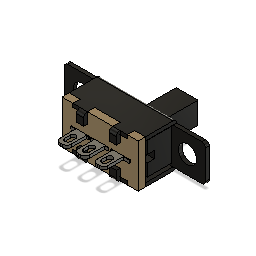
Mini Slide Switch (Autodesk Fusion 360 design; units mm, degrees)
Autodesk Fusion 360 part; units mm, degrees
sketch "Sketch1" plane through (0, 0, 0) normal (0, 1, 0) x (1, 0, 0)
  line L0 (5.25, 2.65) -> (-5.25, 2.65)
  line L1 (-5.25, 2.15) -> (-5.25, -2.65)
  line L2 (-5.25, -2.65) -> (5.25, -2.65)
  line L3 (5.25, -2.65) -> (5.25, 2.15)
  line L4 (5.25, 2.65) -> (-5.25, -2.65) construction
  line L5 (-5.25, 2.65) -> (5.25, -2.65) construction
  line L6 (0, 2.65) -> (9.75, 2.65)
  line L7 (9.75, 2.65) -> (9.75, 2.15)
  line L8 (9.75, 2.15) -> (5.25, 2.15)
  line L9 (0, 2.65) -> (-9.75, 2.65)
  line L10 (-9.75, 2.65) -> (-9.75, 2.15)
  line L11 (-9.75, 2.15) -> (-5.25, 2.15)
  dimension "d1" = 10.5
  dimension "d2" = 5.3
  dimension "d3" = 9.75
  dimension "d4" = 0.5
  dimension "d5" = 9.75
  dimension "d6" = 0.5
  constraint horizontal L0
  constraint perpendicular L0 L1
  constraint parallel L0 L2
  constraint parallel L1 L3
  constraint coincident L4 origin
  constraint coincident L5 origin
  constraint midpoint L0 L6.start
  constraint parallel L0 L6
  constraint perpendicular L6 L7
  constraint perpendicular L3 L8
  constraint parallel L0 L9
  constraint perpendicular L9 L10
  constraint perpendicular L1 L11
  measures "d1" distance of L1.end L2.end
  measures "d2" distance of L0.end L1.end
  measures "d3" distance of L6.start L6.end
  measures "d4" distance of L6.end L7.end
  measures "d5" distance of L6.start L9.end
  measures "d6" distance of L9.end L10.end
extrude "Extrude1" add sketch "Sketch1" along normal blind 6 makes body 1
sketch "Sketch2" plane through (0, 0, -2.65) normal (0, 0, -1) x (-1, 0, 0)
  line L0 (-9.75, 0) -> (9.75, 0)
  line L1 (9.75, 0) -> (9.75, 6)
  line L2 (9.75, 6) -> (-9.75, 6)
  line L3 (-9.75, 6) -> (-9.75, 0)
  line L4 (9.75, 3) -> (7.25, 3)
  line L5 (-9.75, 3) -> (-7.25, 3)
  circle A0 centre (7.25, 3) radius 1.25
  circle A1 centre (-7.25, 3) radius 1.25
  dimension "d9" = 2.5
  dimension "d10" = 2.5
  dimension "d11" = 2.5
  dimension "d12" = 2.5
  constraint midpoint L1 L4.start
  constraint perpendicular L1 L4
  constraint midpoint L3 L5.start
  constraint perpendicular L3 L5
  constraint coincident L4.end A0.centre
  constraint coincident L5.end A1.centre
  measures "d9" distance of L4.start L4.end
  measures "d10" distance of L5.start L5.end
  measures "d11" diameter of A0
  measures "d12" diameter of A1
extrude "Extrude2" cut sketch "Sketch2" against normal blind 5 contours A0 | A1 bodies 1
sketch "Sketch3" plane through (5.25, 0, 0) normal (1, 0, 0) x (0, 0, -1)
  line L0 (-2.65, 0) -> (2.15, 0)
  line L1 (2.15, 0) -> (2.15, 6)
  line L2 (2.15, 6) -> (-2.65, 6)
  line L3 (-2.65, 6) -> (-2.65, 0)
  line L4 (2.15, 5.5) -> (-2.65, 5.5)
  line L5 (-2.65, 0.5) -> (2.15, 0.5)
  constraint coincident L1 L5.end
  constraint coincident L1 L4.start
  constraint coincident L3 L4.end
  constraint coincident L3 L5.start
extrude "Extrude3" cut sketch "Sketch3" against normal blind 16 contours L1 L3 L4 L5 bodies 1
sketch "Sketch4" plane through (0, 0, -2.15) normal (0, 0, 1) x (1, 0, 0)
  circle A0 centre (-7.25, 3) radius 1.25
  circle A1 centre (7.25, 3) radius 1.25
  line L0 (5.25, 0) -> (9.75, 0)
  line L1 (9.75, 0) -> (9.75, 6)
  line L2 (9.75, 6) -> (5.25, 6)
  line L3 (5.25, 6) -> (5.25, 5.5)
  line L4 (5.25, 5.5) -> (-5.25, 5.5)
  line L5 (-5.25, 5.5) -> (-5.25, 6)
  line L6 (-5.25, 6) -> (-9.75, 6)
  line L7 (-9.75, 6) -> (-9.75, 0)
  line L8 (-9.75, 0) -> (-5.25, 0)
  line L9 (-5.25, 0) -> (-5.25, 0.5)
  line L10 (-5.25, 0.5) -> (5.25, 0.5)
  line L11 (5.25, 0.5) -> (5.25, 0)
  line L12 (5.25, 0.5) -> (9.75, 0.5)
  line L13 (5.25, 5.5) -> (9.75, 5.5)
  line L14 (-5.25, 0.5) -> (-9.75, 0.5)
  line L15 (-5.25, 5.5) -> (-9.75, 5.5)
  constraint coincident L10.end L11.start
  constraint coincident L1 L12.end
  constraint perpendicular L1 L12
  constraint coincident L3.end L4.start
  constraint coincident L1 L13.end
  constraint perpendicular L1 L13
  constraint coincident L9.end L10.start
  constraint coincident L7 L14.end
  constraint perpendicular L7 L14
  constraint coincident L4.end L5.start
  constraint coincident L7 L15.end
  constraint perpendicular L7 L15
extrude "Extrude4" cut sketch "Sketch4" against normal blind 15 contours L0 L1 L11 L12 | L7 L8 L9 L14 | L1 L2 L3 L13 | L5 L6 L7 L15 bodies 1
fillet "Fillet2" radius 0.5 4 edges at (-9.75, 0.5, -2.4) (-9.75, 5.5, -2.4) (9.75, 0.5, -2.4) (9.75, 5.5, -2.4) on bodies 1
fillet "Fillet3" radius 0.5 2 edges at (0, 0, -2.65) (0, 6, -2.65) on bodies 1
sketch "Sketch5" plane through (0, 0, -2.65) normal (0, 0, -1) x (-1, 0, 0)
  line L0 (5.25, 5.5) -> (-5.25, 5.5)
  line L1 (-5.25, 5.5) -> (-9.25, 5.5)
  arc A0 (-9.25, 5.5) -> (-9.75, 5) centre (-9.25, 5) ccw
  line L2 (-9.75, 5) -> (-9.75, 1)
  arc A1 (-9.75, 1) -> (-9.25, 0.5) centre (-9.25, 1) ccw
  line L3 (-9.25, 0.5) -> (-5.25, 0.5)
  line L4 (-5.25, 0.5) -> (5.25, 0.5)
  line L5 (5.25, 0.5) -> (9.25, 0.5)
  arc A2 (9.25, 0.5) -> (9.75, 1) centre (9.25, 1) ccw
  line L6 (9.75, 1) -> (9.75, 5)
  arc A3 (9.75, 5) -> (9.25, 5.5) centre (9.25, 5) ccw
  line L7 (9.25, 5.5) -> (5.25, 5.5)
  circle A4 centre (7.25, 3) radius 1.25
  circle A5 centre (-7.25, 3) radius 1.25
  line L8 (-3, 1.5) -> (3, 1.5)
  line L9 (3, 1.5) -> (3, 4.5)
  line L10 (3, 4.5) -> (-3, 4.5)
  line L11 (-3, 4.5) -> (-3, 1.5)
  line L12 (-3, 1.5) -> (3, 4.5) construction
  line L13 (3, 1.5) -> (-3, 4.5) construction
  point P0 (0, 3)
  dimension "d26" = 6
  dimension "d27" = 3
  constraint horizontal L8
  constraint perpendicular L8 L9
  constraint parallel L8 L10
  constraint parallel L9 L11
  constraint coincident L12 P0
  constraint coincident L13 P0
  measures "d26" distance of L9.end L10.end
  measures "d27" distance of L8.end L9.end
extrude "Extrude5" cut sketch "Sketch5" against normal blind 4 contours L8 L9 L10 L11 bodies 1
sketch "Sketch6" plane through (0, 0, 0) normal (0, -1, 0) x (1, 0, 0)
  line L0 (-5.25, -2.15) -> (5.25, -2.15)
  line L1 (5.25, -2.15) -> (5.25, 2.65)
  line L2 (5.25, 2.65) -> (-5.25, 2.65)
  line L3 (-5.25, 2.65) -> (-5.25, -2.15)
  line L4 (5.25, 2.65) -> (3.75, 2.65)
  line L5 (3.75, 2.65) -> (3.75, 1.65)
  line L6 (3.75, 1.65) -> (5.25, 1.65)
  line L7 (-5.25, 2.65) -> (-5.25, 1.65)
  line L8 (-5.25, 1.65) -> (-3.75, 1.65)
  line L9 (3.75, 2.65) -> (1.75, 2.65)
  line L10 (1.75, 2.65) -> (1.75, 1.65)
  line L11 (-3.75, 1.65) -> (-3.75, 2.65)
  line L12 (-3.75, 2.65) -> (-1.75, 2.65)
  line L13 (-1.75, 2.65) -> (-1.75, 1.65)
  line L14 (1.75, 1.65) -> (-1.75, 1.65)
  dimension "d30" = 1.5
  dimension "d31" = 1
  dimension "d32" = 1
  dimension "d33" = 1.5
  dimension "d34" = 2
  dimension "d35" = 1
  dimension "d36" = 2
  dimension "d37" = 1
  constraint coincident L1.end L2.start
  constraint perpendicular L1 L4
  constraint perpendicular L4 L5
  constraint coincident L1 L6.end
  constraint perpendicular L1 L6
  constraint coincident L2.end L3.start
  constraint perpendicular L2 L7
  constraint perpendicular L3 L8
  constraint perpendicular L5 L9
  constraint perpendicular L9 L10
  constraint coincident L2 L11.end
  constraint perpendicular L2 L11
  constraint perpendicular L11 L12
  constraint perpendicular L2 L13
  measures "d30" distance of L1.end L4.end
  measures "d31" distance of L4.end L5.end
  measures "d32" distance of L2.end L7.end
  measures "d33" distance of L7.end L8.end
  measures "d34" distance of L4.end L9.end
  measures "d35" distance of L9.end L10.end
  measures "d36" distance of L11.end L12.end
  measures "d37" distance of L12.end L13.end
extrude "Extrude6" cut sketch "Sketch6" against normal blind 11 contours L2 L3 L7 L8 L11 | L1 L2 L4 L5 L6 | L2 L10 L13 L14 bodies 1
sketch "Sketch7" plane through (0, 0, 1.65) normal (0, 0, 1) x (1, 0, 0)
  line L0 (-3.75, 0.5) -> (-5.25, 0.5)
  line L1 (-5.25, 0.5) -> (-5.25, 0)
  line L2 (-5.25, 0) -> (-3.75, 0)
  line L3 (-3.75, 0) -> (-3.75, 0.5)
  line L4 (-5.25, 0) -> (5.25, 0)
  line L5 (5.25, 0) -> (5.25, 6)
  line L6 (5.25, 6) -> (-5.25, 6)
  line L7 (-5.25, 6) -> (-5.25, 0)
  line L8 (-3.75, 0) -> (-1.75, 0)
  line L9 (-1.75, 0) -> (-1.75, 0.5)
  line L10 (-1.75, 0.5) -> (-3.75, 0.5)
  line L11 (-3.75, 0.5) -> (-3.75, 0)
  line L12 (0, 0) -> (0, 6)
  line L13 (-5.25, 3) -> (5.25, 3)
  line L14 (-1.75, 6) -> (-1.75, 5.5)
  line L15 (-1.75, 5.5) -> (-3.75, 5.5)
  line L16 (-3.75, 5.5) -> (-3.75, 6)
  line L17 (1.75, 0.5) -> (3.75, 0.5)
  line L18 (1.75, 0) -> (1.75, 0.5)
  line L19 (3.75, 0.5) -> (3.75, 0)
  line L20 (1.75, 5.5) -> (3.75, 5.5)
  line L21 (1.75, 6) -> (1.75, 5.5)
  line L22 (3.75, 5.5) -> (3.75, 6)
  dimension "d40" = 10.5
  dimension "d41" = 6
  dimension "d42" = 2
  constraint horizontal L4
  constraint vertical L5
  constraint horizontal L6
  constraint vertical L7
  constraint coincident L1.end L2.start
  constraint horizontal L8
  constraint vertical L9
  constraint horizontal L10
  constraint vertical L11
  constraint coincident L2.end L3.start
  constraint coincident L12.start origin
  constraint midpoint L6 L12.end
  constraint midpoint L7 L13.start
  constraint midpoint L5 L13.end
  constraint symmetric L2.end L13 L16.end
  constraint symmetric L8.end L13 L14.start
  constraint symmetric L9.end L13 L14.end
  constraint symmetric L0.start L13 L15.end
  constraint symmetric L2.end L12 L19.end
  constraint symmetric L8.end L12 L18.start
  constraint symmetric L9.end L12 L17.start
  constraint symmetric L0.start L12 L17.end
  constraint symmetric L12 L14.start L21.start
  constraint symmetric L12 L14.end L20.start
  constraint symmetric L12 L15.end L20.end
  constraint symmetric L12 L16.end L22.end
  measures "d40" distance of L1.end L4.end
  measures "d41" distance of L1.end L6.end
  measures "d42" distance of L2.end L8.end
extrude "Extrude7" add sketch "Sketch7" along normal blind 1 separate body contours L0 L1 L2 L3 L4 L7 L11 | L0 L4 L7 L9 L10 L12 L13 | L6 L7 L12 L13 L14 L15 L16 | L4 L5 L12 L13 L17 L18 L19 | L5 L6 L12 L13 L20 L21 L22 makes body 2
sketch "Sketch8" plane through (0, 0, 2.65) normal (0, 0, 1) x (1, 0, 0)
  line L0 (-1.75, 0) -> (-1.75, 0.5)
  line L1 (-1.75, 0.5) -> (-3.75, 0.5)
  line L2 (-3.75, 0.5) -> (-3.75, 0)
  line L3 (-3.75, 0) -> (-1.75, 0)
  line L4 (-1.75, 0) -> (-2.75, 0)
  line L5 (-2.75, 0) -> (-2.75, 1.5)
  line L6 (-2.75, 1.5) -> (-1.75, 1.5)
  line L7 (-1.75, 1.5) -> (-1.75, 0)
  line L8 (0, 0) -> (0, 6)
  line L9 (0, 3) -> (-5, 3)
  line L10 (-1.75, 4.5) -> (-1.75, 6)
  line L11 (-2.75, 4.5) -> (-1.75, 4.5)
  line L12 (-2.75, 6) -> (-2.75, 4.5)
  line L13 (-1.75, 6) -> (-2.75, 6)
  line L14 (1.75, 1.5) -> (1.75, 0)
  line L15 (2.75, 1.5) -> (1.75, 1.5)
  line L16 (2.75, 0) -> (2.75, 1.5)
  line L17 (1.75, 0) -> (2.75, 0)
  line L18 (2.75, 4.5) -> (1.75, 4.5)
  line L19 (1.75, 4.5) -> (1.75, 6)
  line L20 (2.75, 6) -> (2.75, 4.5)
  line L21 (1.75, 6) -> (2.75, 6)
  dimension "d45" = 1.5
  constraint horizontal L4
  constraint vertical L5
  constraint horizontal L6
  constraint vertical L7
  constraint coincident L0.start L3.end
  constraint coincident L8.start origin
  constraint vertical L8
  constraint midpoint L8 L9.start
  constraint perpendicular L8 L9
  constraint symmetric L0.start L9 L10.end
  constraint symmetric L4.end L9 L12.start
  constraint symmetric L5.end L9 L11.start
  constraint symmetric L6.end L9 L10.start
  constraint symmetric L0.start L8 L14.end
  constraint symmetric L4.end L8 L16.start
  constraint symmetric L5.end L8 L15.start
  constraint symmetric L6.end L8 L14.start
  constraint symmetric L8 L10.start L18.end
  constraint symmetric L8 L10.end L19.end
  constraint symmetric L8 L11.start L18.start
  constraint symmetric L8 L12.start L20.start
  measures "d45" distance of L0.start L6.end
extrude "Extrude8" add sketch "Sketch8" along normal blind 0.5 contours L0 L1 L3 L4 L5 L7 | L1 L5 L6 L7 | L10 L11 L12 L13 | L14 L15 L16 L17 | L18 L19 L20 L21 bodies 1
fillet "Fillet4" radius 0.5 4 edges at (-2.25, 0, 3.15) (2.25, 0, 3.15) (2.25, 6, 3.15) (-2.25, 6, 3.15) on bodies 1
sketch "Sketch9" plane through (0, 0, 1.65) normal (0, 0, -1) x (-1, 0, 0)
  line L0 (1.75, 6) -> (-1.75, 6)
  line L1 (-1.75, 6) -> (-1.75, 5.5)
  line L2 (-1.75, 5.5) -> (-3.75, 5.5)
  line L3 (-3.75, 5.5) -> (-3.75, 6)
  line L4 (-3.75, 6) -> (-5.25, 6)
  line L5 (-5.25, 6) -> (-5.25, 0)
  line L6 (-5.25, 0) -> (-3.75, 0)
  line L7 (-3.75, 0) -> (-3.75, 0.5)
  line L8 (-3.75, 0.5) -> (-1.75, 0.5)
  line L9 (-1.75, 0.5) -> (-1.75, 0)
  line L10 (-1.75, 0) -> (1.75, 0)
  line L11 (1.75, 0) -> (1.75, 0.5)
  line L12 (1.75, 0.5) -> (3.75, 0.5)
  line L13 (3.75, 0.5) -> (3.75, 0)
  line L14 (3.75, 0) -> (5.25, 0)
  line L15 (5.25, 0) -> (5.25, 6)
  line L16 (5.25, 6) -> (3.75, 6)
  line L17 (3.75, 6) -> (3.75, 5.5)
  line L18 (3.75, 5.5) -> (1.75, 5.5)
  line L19 (1.75, 5.5) -> (1.75, 6)
  line L20 (0, 0) -> (0, 6)
  line L21 (5.25, 3) -> (-5.25, 3)
  line L22 (-1.2, 2.8) -> (1.2, 2.8)
  line L23 (1.2, 2.8) -> (1.2, 3.2)
  line L24 (1.2, 3.2) -> (-1.2, 3.2)
  line L25 (-1.2, 3.2) -> (-1.2, 2.8)
  line L26 (-1.2, 2.8) -> (1.2, 3.2) construction
  line L27 (1.2, 2.8) -> (-1.2, 3.2) construction
  line L28 (0, 3) -> (-2.54, 3)
  line L29 (-0.0656, 3) -> (2.4744, 3)
  line L30 (1.4744, 2.8) -> (3.4744, 2.8)
  line L31 (3.4744, 2.8) -> (3.4744, 3.2)
  line L32 (3.4744, 3.2) -> (1.4744, 3.2)
  line L33 (1.4744, 3.2) -> (1.4744, 2.8)
  line L34 (1.4744, 2.8) -> (3.4744, 3.2) construction
  line L35 (3.4744, 2.8) -> (1.4744, 3.2) construction
  line L36 (-3.54, 2.8) -> (-1.54, 2.8)
  line L37 (-1.54, 2.8) -> (-1.54, 3.2)
  line L38 (-1.54, 3.2) -> (-3.54, 3.2)
  line L39 (-3.54, 3.2) -> (-3.54, 2.8)
  line L40 (-3.54, 2.8) -> (-1.54, 3.2) construction
  line L41 (-1.54, 2.8) -> (-3.54, 3.2) construction
  line L42 (0, 3) -> (-4.25, 3)
  line L43 (-1.54, 3.2) -> (-4.14, 3.2)
  line L44 (-1.54, 2.8) -> (-4.14, 2.8)
  line L45 (-4.14, 2.8) -> (-4.14, 3.2)
  line L46 (1.4744, 2.8) -> (3.9744, 2.8)
  line L47 (3.9744, 2.8) -> (3.9744, 3.2)
  line L48 (3.9744, 3.2) -> (3.4744, 3.2)
  point P0 (0, 3)
  point P1 (2.4744, 3)
  point P2 (-2.54, 3)
  dimension "d57" = 2.4
  dimension "d58" = 0.4
  dimension "d59" = 2.54
  dimension "d60" = 2.54
  dimension "d61" = 2
  dimension "d62" = 2
  dimension "d63" = 0.4
  dimension "d64" = 4.25
  dimension "d65" = 2.6
  dimension "d66" = 2.5
  constraint coincident L20.start origin
  constraint midpoint L0 L20.end
  constraint midpoint L15 L21.start
  constraint midpoint L5 L21.end
  constraint horizontal L22
  constraint perpendicular L22 L23
  constraint parallel L22 L24
  constraint parallel L23 L25
  constraint coincident L26 P0
  constraint coincident L27 P0
  constraint midpoint L20 P0
  constraint coincident P0 L28.start
  constraint parallel L21 L28
  constraint coincident L21 L29.start
  constraint perpendicular L23 L29
  constraint horizontal L30
  constraint perpendicular L30 L31
  constraint parallel L30 L32
  constraint parallel L31 L33
  constraint coincident L34 P1
  constraint coincident L35 P1
  constraint coincident P1 L29.end
  constraint horizontal L36
  constraint perpendicular L36 L37
  constraint parallel L36 L38
  constraint parallel L37 L39
  constraint coincident L40 P2
  constraint coincident L41 P2
  constraint coincident P2 L28.end
  constraint perpendicular L39 L42
  constraint perpendicular L39 L43
  constraint perpendicular L37 L44
  constraint perpendicular L43 L45
  constraint perpendicular L31 L46
  constraint perpendicular L21 L47
  constraint perpendicular L31 L48
  measures "d57" distance of L23.end L24.end
  measures "d58" distance of L22.end L23.end
  measures "d59" distance of P0 P2
  measures "d60" distance of L29.start P1
  measures "d61" distance of L31.end L32.end
  measures "d62" distance of L37.end L38.end
  measures "d63" distance of L36.end L37.end
  measures "d64" distance of P0 L42.end
  measures "d65" distance of L37.end L43.end
  measures "d66" distance of L30.start L46.end
extrude "Extrude9" cut sketch "Sketch9" against normal blind 2 contours L20 L21 L23 L24 L29 | L20 L21 L24 L25 L28 L29 L42 | L20 L21 L22 L23 L29 | L20 L21 L22 L25 L28 L29 L42 | L21 L29 L31 L32 L33 | L21 L29 L30 L31 L33 L46 | L21 L28 L36 L37 L39 L42 L44 | L21 L28 L37 L38 L39 L42 L43 | L21 L31 L46 L47 | L21 L31 L47 L48 | L21 L39 L42 L44 L45 | L21 L39 L42 L43 L45 bodies 2
sketch "Sketch10" plane through (0, 0, 1.65) normal (0, 0, -1) x (-1, 0, 0)
  line L0 (1.4744, 2.8) -> (1.4744, 3.2)
  line L1 (1.4744, 3.2) -> (3.9744, 3.2)
  line L2 (3.9744, 3.2) -> (3.9744, 2.8)
  line L3 (3.9744, 2.8) -> (1.4744, 2.8)
  line L4 (1.2, 2.8) -> (-1.2, 2.8)
  line L5 (-1.2, 2.8) -> (-1.2, 3.2)
  line L6 (-1.2, 3.2) -> (1.2, 3.2)
  line L7 (1.2, 3.2) -> (1.2, 2.8)
  line L8 (-4.14, 3.2) -> (-1.54, 3.2)
  line L9 (-1.54, 3.2) -> (-1.54, 2.8)
  line L10 (-1.54, 2.8) -> (-4.14, 2.8)
  line L11 (-4.14, 2.8) -> (-4.14, 3.2)
  line L12 (1.75, 6) -> (-1.75, 6)
  line L13 (-1.75, 6) -> (-1.75, 5.5)
  line L14 (-1.75, 5.5) -> (-3.75, 5.5)
  line L15 (-3.75, 5.5) -> (-3.75, 6)
  line L16 (-3.75, 6) -> (-5.25, 6)
  line L17 (-5.25, 6) -> (-5.25, 0)
  line L18 (-5.25, 0) -> (-3.75, 0)
  line L19 (-3.75, 0) -> (-3.75, 0.5)
  line L20 (-3.75, 0.5) -> (-1.75, 0.5)
  line L21 (-1.75, 0.5) -> (-1.75, 0)
  line L22 (-1.75, 0) -> (1.75, 0)
  line L23 (1.75, 0) -> (1.75, 0.5)
  line L24 (1.75, 0.5) -> (3.75, 0.5)
  line L25 (3.75, 0.5) -> (3.75, 0)
  line L26 (3.75, 0) -> (5.25, 0)
  line L27 (5.25, 0) -> (5.25, 6)
  line L28 (5.25, 6) -> (3.75, 6)
  line L29 (3.75, 6) -> (3.75, 5.5)
  line L30 (3.75, 5.5) -> (1.75, 5.5)
  line L31 (1.75, 5.5) -> (1.75, 6)
extrude "Extrude10" add sketch "Sketch10" along normal blind 1 and the other way blind 1.1 separate body contours L0 L1 L2 L3 | L4 L5 L6 L7 | L8 L9 L10 L11 makes body 3 at (-2.3078, 2.8, 1.35) makes body 4 at (0.4, 2.8, 1.35) makes body 5 at (2.4067, 2.8, 2.05)
extrude "Extrude11" cut 2 faces at (-2.3078, 3.0667, 0.65) (3.2733, 3.0667, 0.65) along direction (0, 0, 1) blind 0.2 on bodies 3 5 bodies 3 5
sketch "Sketch11" plane through (0, 3.2, 0) normal (0, 1, 0) x (-1, 0, 0)
  line L0 (-1.2, 2.75) -> (-1.2, 0.65)
  line L1 (-1.2, 0.65) -> (1.2, 0.65)
  line L2 (1.2, 0.65) -> (1.2, 2.75)
  line L3 (1.2, 2.75) -> (-1.2, 2.75)
  line L4 (1.2, 0.65) -> (1.2, 0.85)
  line L5 (1.2, 0.85) -> (-1.2, 0.85)
  arc A0 (-1.2, 0.85) -> (1.2, 0.85) centre (0, 4.35) ccw
  dimension "d75" = 0.2
  constraint coincident L1.end L2.start
  constraint perpendicular L1 L4
  constraint coincident L0 L5.end
  constraint perpendicular L0 L5
  measures "d75" distance of L1.end L4.end
extrude "Extrude12" cut sketch "Sketch11" against normal blind 1.3 contours L0 L1 A0 | L1 L2 L4 A0 bodies 4
sketch "Sketch12" plane through (0, 0, 2.75) normal (0, 0, 1) x (1, 0, 0)
  line L0 (1.2, 3.2) -> (-1.2, 3.2)
  line L1 (-1.2, 3.2) -> (-1.2, 2.8)
  line L2 (-1.2, 2.8) -> (1.2, 2.8)
  line L3 (1.2, 2.8) -> (1.2, 3.2)
  line L4 (0.75, 3.2) -> (-0.75, 3.2)
  line L5 (-0.75, 3.2) -> (-0.75, 2.8)
  line L6 (-0.75, 2.8) -> (0.75, 2.8)
  line L7 (0.75, 2.8) -> (0.75, 3.2)
  line L8 (0.75, 3.2) -> (-0.75, 2.8) construction
  line L9 (-0.75, 3.2) -> (0.75, 2.8) construction
  line L10 (0, 3) -> (2.54, 3)
  line L11 (0, 3) -> (-2.54, 3)
  line L12 (3.29, 3.2) -> (1.79, 3.2)
  line L13 (1.79, 3.2) -> (1.79, 2.8)
  line L14 (1.79, 2.8) -> (3.29, 2.8)
  line L15 (3.29, 2.8) -> (3.29, 3.2)
  line L16 (3.29, 3.2) -> (1.79, 2.8) construction
  line L17 (1.79, 3.2) -> (3.29, 2.8) construction
  line L18 (-1.79, 3.2) -> (-3.29, 3.2)
  line L19 (-3.29, 3.2) -> (-3.29, 2.8)
  line L20 (-3.29, 2.8) -> (-1.79, 2.8)
  line L21 (-1.79, 2.8) -> (-1.79, 3.2)
  line L22 (-1.79, 3.2) -> (-3.29, 2.8) construction
  line L23 (-3.29, 3.2) -> (-1.79, 2.8) construction
  point P0 (0, 3)
  point P1 (2.54, 3)
  point P2 (-2.54, 3)
  dimension "d78" = 1.5
  dimension "d79" = 2.54
  dimension "d80" = 2.54
  dimension "d81" = 1.5
  dimension "d82" = 1.5
  constraint horizontal L4
  constraint perpendicular L4 L5
  constraint parallel L4 L6
  constraint parallel L5 L7
  constraint coincident L8 P0
  constraint coincident L9 P0
  constraint coincident P0 L10.start
  constraint parallel L0 L10
  constraint parallel L10 L11
  constraint horizontal L12
  constraint perpendicular L12 L13
  constraint parallel L12 L14
  constraint parallel L13 L15
  constraint coincident L16 P1
  constraint coincident L17 P1
  constraint coincident P1 L10.end
  constraint horizontal L18
  constraint perpendicular L18 L19
  constraint parallel L18 L20
  constraint parallel L19 L21
  constraint coincident L22 P2
  constraint coincident L23 P2
  constraint coincident P2 L11.end
  measures "d78" distance of L5.end L6.end
  measures "d79" distance of P0 P1
  measures "d80" distance of P0 P2
  measures "d81" distance of L13.end L14.end
  measures "d82" distance of L19.end L20.end
extrude "Extrude13" add sketch "Sketch12" along normal blind 2.7 contours L0 L4 L5 L7 L10 L11 | L2 L5 L6 L7 L10 L11 | L12 L13 L14 L15 | L18 L19 L20 L21 bodies 3 4 5
fillet "Fillet5" radius 0.6 6 edges at (-1.79, 3, 5.45) (-3.29, 3, 5.45) (-0.75, 3, 5.45) (0.75, 3, 5.45) (1.79, 3, 5.45) (3.29, 3, 5.45) on bodies 3 4 5
sketch "Sketch13" plane through (0, 2.8, 0) normal (0, -1, 0) x (1, 0, 0)
  arc A0 (0.75, 4.85) -> (0.15, 5.45) centre (0.15, 4.85) ccw
  line L0 (0.15, 5.45) -> (-0.15, 5.45)
  arc A1 (-0.15, 5.45) -> (-0.75, 4.85) centre (-0.15, 4.85) ccw
  line L1 (-0.75, 4.85) -> (-0.75, 2.75)
  line L2 (-0.75, 2.75) -> (-1.2, 2.75)
  line L3 (-1.2, 2.75) -> (-1.2, 0.85)
  arc A2 (-1.2, 0.85) -> (1.2, 0.85) centre (0, 4.35) ccw
  line L4 (1.2, 0.85) -> (1.2, 2.75)
  line L5 (1.2, 2.75) -> (0.75, 2.75)
  line L6 (0.75, 2.75) -> (0.75, 4.85)
  line L7 (0, 5.45) -> (0, 4.95)
  line L8 (0, 4.95) -> (0, 3.45)
  line L9 (-0.4, 4.55) -> (-0.4025, 3.8514)
  line L10 (0.4, 4.55) -> (0.3975, 3.8486)
  arc A3 (0.4, 4.5472) -> (-0.4, 4.55) centre (0, 4.55) ccw
  arc A4 (-0.4025, 3.8514) -> (0.3975, 3.8486) centre (-0.0025, 3.85) ccw
  line L11 (0, 4.55) -> (2.54, 4.55)
  line L12 (1.27, 4.55) -> (1.27, 3.7407)
  arc A5 (2.94, 4.55) -> (2.14, 4.5472) centre (2.54, 4.55) ccw
  line L13 (2.94, 4.55) -> (2.9425, 3.8514)
  arc A6 (2.1425, 3.8486) -> (2.9425, 3.8514) centre (2.5425, 3.85) ccw
  line L14 (2.14, 4.55) -> (2.1425, 3.8486)
  line L15 (-2.14, 4.55) -> (-2.1425, 3.8486)
  arc A7 (-2.9425, 3.8514) -> (-2.1425, 3.8486) centre (-2.5425, 3.85) ccw
  line L16 (-2.94, 4.55) -> (-2.9425, 3.8514)
  arc A8 (-2.14, 4.5472) -> (-2.94, 4.55) centre (-2.54, 4.55) ccw
  dimension "d88" = 0.5
  dimension "d89" = 0.8
  dimension "d90" = 1.5
  dimension "d91" = 0.8
  dimension "d92" = 2.54
  constraint midpoint L0 L7.start
  constraint perpendicular L0 L7
  constraint coincident L7.end A3
  constraint parallel L7 L8
  constraint coincident L8.end A4
  constraint tangent L9 A4
  constraint coincident L10.start A3
  constraint tangent L10 A4
  constraint coincident L10 A3.start
  constraint coincident A3.centre L11.start
  constraint perpendicular L8 L11
  constraint midpoint L11 L12.start
  constraint perpendicular L11 L12
  constraint symmetric L9.start L12 A5.start
  constraint symmetric L9.end L12 L13.end
  constraint symmetric L10.start L12 L14.start
  constraint symmetric L10.end L12 A6.start
  constraint symmetric A3.start L12 A5.end
  constraint symmetric A3 L12 A5
  constraint symmetric A4 L12 A6
  constraint symmetric L7 A5.end A8.start
  constraint symmetric L7 A5.start L16.start
  constraint symmetric L7 A5 A8
  constraint symmetric L7 L13.end A7.start
  constraint symmetric L7 A6.start L15.end
  constraint symmetric L7 A6 A7
  constraint symmetric L7 L14.start L15.start
  measures "d88" distance of L7.start L7.end
  measures "d89" diameter of A3
  measures "d90" distance of L7.end L8.end
  measures "d91" diameter of A4
  measures "d92" distance of A3.centre L11.end
extrude "Extrude14" cut sketch "Sketch13" against normal blind 1 contours L8 A3 L11 | L8 L10 A3 A4 L11 | L8 L9 A3 A4 | A5 L13 A6 L14 | L15 A7 L16 A8 bodies 3 4 5
sketch "Sketch14" plane through (0, 0, -2.15) normal (0, 0, 1) x (1, 0, 0)
  line L0 (3, 1.5) -> (-3, 1.5)
  line L1 (-3, 1.5) -> (-3, 4.5)
  line L2 (-3, 4.5) -> (3, 4.5)
  line L3 (3, 4.5) -> (3, 1.5)
  arc A0 (9.75, 5) -> (9.25, 5.5) centre (9.25, 5) ccw
  line L4 (9.25, 5.5) -> (5.25, 5.5)
  line L5 (5.25, 5.5) -> (-5.25, 5.5)
  line L6 (-5.25, 5.5) -> (-9.25, 5.5)
  arc A1 (-9.25, 5.5) -> (-9.75, 5) centre (-9.25, 5) ccw
  line L7 (-9.75, 5) -> (-9.75, 1)
  arc A2 (-9.75, 1) -> (-9.25, 0.5) centre (-9.25, 1) ccw
  line L8 (-9.25, 0.5) -> (-5.25, 0.5)
  line L9 (-5.25, 0.5) -> (5.25, 0.5)
  line L10 (5.25, 0.5) -> (9.25, 0.5)
  arc A3 (9.25, 0.5) -> (9.75, 1) centre (9.25, 1) ccw
  line L11 (9.75, 1) -> (9.75, 5)
  circle A4 centre (-7.25, 3) radius 1.25
  circle A5 centre (7.25, 3) radius 1.25
  line L12 (0, 1.5) -> (0, 4.5)
  line L13 (0, 3) -> (3, 3)
  line L14 (5, 5.2) -> (-2, 5.2)
  line L15 (-2, 5.2) -> (-2, 0.8)
  line L16 (-2, 0.8) -> (5, 0.8)
  line L17 (5, 0.8) -> (5, 5.2)
  line L18 (5, 5.2) -> (-2, 0.8) construction
  line L19 (-2, 5.2) -> (5, 0.8) construction
  point P0 (1.5, 3)
  dimension "d95" = 7
  dimension "d96" = 4.4
  constraint midpoint L0 L12.start
  constraint midpoint L2 L12.end
  constraint midpoint L12 L13.start
  constraint midpoint L3 L13.end
  constraint horizontal L14
  constraint perpendicular L14 L15
  constraint parallel L14 L16
  constraint parallel L15 L17
  constraint coincident L18 P0
  constraint coincident L19 P0
  constraint midpoint L13 P0
  measures "d95" distance of L15.end L16.end
  measures "d96" distance of L14.end L15.end
extrude "Extrude15" add sketch "Sketch14" along normal blind 3.3 separate body contours L0 L2 L3 L14 L15 L16 L17 | L0 L3 L12 L13 | L0 L2 L12 L15 | L2 L3 L12 L13 makes body 6
sketch "Sketch15" plane through (0, 0, -2.15) normal (0, 0, -1) x (-1, 0, 0)
  line L0 (-5, 5.2) -> (-5, 0.8)
  line L1 (-5, 0.8) -> (2, 0.8)
  line L2 (2, 0.8) -> (2, 5.2)
  line L3 (2, 5.2) -> (-5, 5.2)
  line L4 (2, 3) -> (-5, 3)
  line L5 (-3, 1.5) -> (0, 1.5)
  line L6 (0, 1.5) -> (0, 4.5)
  line L7 (0, 4.5) -> (-3, 4.5)
  line L8 (-3, 4.5) -> (-3, 1.5)
  line L9 (-3, 1.5) -> (0, 4.5) construction
  line L10 (0, 1.5) -> (-3, 4.5) construction
  point P0 (-1.5, 3)
  dimension "d99" = 3
  dimension "d100" = 3
  constraint midpoint L2 L4.start
  constraint midpoint L0 L4.end
  constraint horizontal L5
  constraint perpendicular L5 L6
  constraint parallel L5 L7
  constraint parallel L6 L8
  constraint coincident L9 P0
  constraint coincident L10 P0
  constraint midpoint L4 P0
  measures "d99" distance of L6.end L7.end
  measures "d100" distance of L5.end L6.end
extrude "Extrude16" add sketch "Sketch15" along normal blind 5.7 contours L4 L6 L7 L8 | L4 L5 L6 L8 bodies 6
sketch "Sketch16" plane through (0, 5.2, 0) normal (0, 1, 0) x (-1, 0, 0)
  line L0 (-5, -2.15) -> (2, -2.15)
  line L1 (2, -2.15) -> (2, 1.15)
  line L2 (2, 1.15) -> (-5, 1.15)
  line L3 (-5, 1.15) -> (-5, -2.15)
  line L4 (2, 1.15) -> (0.3, 1.15)
  line L5 (0.3, 1.15) -> (0.3, -1.45)
  line L6 (-5, 1.15) -> (-4, 1.15)
  line L7 (-4, 1.15) -> (-4, -1.45)
  line L8 (0.3, -1.45) -> (-4, -1.45)
  dimension "d103" = 1.7
  dimension "d104" = 2.6
  dimension "d105" = 1
  dimension "d106" = 2.6
  constraint coincident L1.end L2.start
  constraint perpendicular L1 L4
  constraint perpendicular L2 L5
  constraint coincident L2.end L3.start
  constraint perpendicular L3 L6
  constraint perpendicular L2 L7
  measures "d103" distance of L1.end L4.end
  measures "d104" distance of L4.end L5.end
  measures "d105" distance of L2.end L6.end
  measures "d106" distance of L6.end L7.end
extrude "Extrude17" cut sketch "Sketch16" against normal blind 0.75 contours L2 L5 L7 L8 bodies 6
sketch "Sketch17" plane through (0, 0.8, 0) normal (0, -1, 0) x (1, 0, 0)
  line L0 (-2, -2.15) -> (5, -2.15)
  line L1 (5, -2.15) -> (5, 1.15)
  line L2 (5, 1.15) -> (-2, 1.15)
  line L3 (-2, 1.15) -> (-2, -2.15)
  line L4 (5, 1.15) -> (3.3, 1.15)
  line L5 (3.3, 1.15) -> (3.3, -1.45)
  line L6 (-2, 1.15) -> (-1, 1.15)
  line L7 (-1, 1.15) -> (-1, -1.45)
  line L8 (3.3, -1.45) -> (-1, -1.45)
  dimension "d109" = 1.7
  dimension "d110" = 2.6
  dimension "d111" = 1
  dimension "d112" = 2.6
  constraint coincident L1.end L2.start
  constraint perpendicular L1 L4
  constraint perpendicular L4 L5
  constraint coincident L2.end L3.start
  constraint perpendicular L3 L6
  constraint perpendicular L6 L7
  measures "d109" distance of L1.end L4.end
  measures "d110" distance of L4.end L5.end
  measures "d111" distance of L2.end L6.end
  measures "d112" distance of L6.end L7.end
extrude "Extrude18" cut sketch "Sketch17" against normal blind 0.75 contours L2 L5 L7 L8 bodies 6
sketch "Sketch18" plane through (0, 0, 1.15) normal (0, 0, 1) x (1, 0, 0)
  line L0 (3.3, 1.55) -> (3.3, 0.8)
  line L1 (3.3, 0.8) -> (5, 0.8)
  line L2 (5, 0.8) -> (5, 5.2)
  line L3 (5, 5.2) -> (4, 5.2)
  line L4 (4, 5.2) -> (4, 4.45)
  line L5 (4, 4.45) -> (-0.3, 4.45)
  line L6 (-0.3, 4.45) -> (-0.3, 5.2)
  line L7 (-0.3, 5.2) -> (-2, 5.2)
  line L8 (-2, 5.2) -> (-2, 0.8)
  line L9 (-2, 0.8) -> (-1, 0.8)
  line L10 (-1, 0.8) -> (-1, 1.55)
  line L11 (-1, 1.55) -> (3.3, 1.55)
  line L12 (5, 3) -> (-2, 3)
  line L13 (-2, 2.5) -> (5, 2.5)
  line L14 (5, 2.5) -> (5, 3.5)
  line L15 (5, 3.5) -> (-2, 3.5)
  line L16 (-2, 3.5) -> (-2, 2.5)
  line L17 (-2, 2.5) -> (5, 3.5) construction
  line L18 (5, 2.5) -> (-2, 3.5) construction
  point P0 (1.5, 3)
  dimension "d115" = 1
  constraint midpoint L2 L12.start
  constraint midpoint L8 L12.end
  constraint horizontal L13
  constraint perpendicular L13 L14
  constraint parallel L13 L15
  constraint parallel L14 L16
  constraint coincident L17 P0
  constraint coincident L18 P0
  constraint midpoint L12 P0
  measures "d115" distance of L13.end L14.end
extrude "Extrude19" cut sketch "Sketch18" against normal blind 1 contours L2 L8 L12 L13 L14 L16 | L2 L8 L12 L14 L15 L16 bodies 6
sketch "Sketch19" plane through (0, 0, 1.15) normal (0, 0, 1) x (1, 0, 0)
  line L0 (-2, 3.5) -> (5, 3.5)
  line L1 (5, 3.5) -> (5, 5.2)
  line L2 (5, 5.2) -> (4, 5.2)
  line L3 (4, 5.2) -> (4, 4.45)
  line L4 (4, 4.45) -> (-0.3, 4.45)
  line L5 (-0.3, 4.45) -> (-0.3, 5.2)
  line L6 (-0.3, 5.2) -> (-2, 5.2)
  line L7 (-2, 5.2) -> (-2, 3.5)
  line L8 (-2, 5.2) -> (-2, 0.8)
  line L9 (-2, 3) -> (5, 3)
  line L10 (4, 4) -> (-1, 4)
  line L11 (-1, 4) -> (-1, 2)
  line L12 (-1, 2) -> (4, 2)
  line L13 (4, 2) -> (4, 4)
  line L14 (4, 4) -> (-1, 2) construction
  line L15 (-1, 4) -> (4, 2) construction
  point P0 (1.5, 3)
  dimension "d118" = 2
  constraint coincident L6.end L7.start
  constraint perpendicular L6 L8
  constraint midpoint L8 L9.start
  constraint perpendicular L8 L9
  constraint horizontal L10
  constraint perpendicular L10 L11
  constraint parallel L10 L12
  constraint parallel L11 L13
  constraint coincident L14 P0
  constraint coincident L15 P0
  constraint midpoint L9 P0
  measures "d118" distance of L10.end L11.end
extrude "Extrude20" cut sketch "Sketch19" against normal blind 2.5 contours L0 L10 L11 L13 | L0 L9 L11 L13 | L9 L11 L12 L13 bodies 6
sketch "Sketch20" plane through (0, 0, -1.35) normal (0, 0, 1) x (1, 0, 0)
  line L0 (4, 2) -> (4, 4)
  line L1 (4, 4) -> (-1, 4)
  line L2 (-1, 4) -> (-1, 2)
  line L3 (-1, 2) -> (4, 2)
  line L4 (-1, 4) -> (4, 2)
  circle A0 centre (1.5, 3) radius 1.1
  constraint coincident L1.end L2.start
  constraint coincident L0.start L3.end
  constraint midpoint L4 A0.centre
extrude "Extrude21" cut sketch "Sketch20" along normal blind 2.9 and the other way blind 1.2 contours L3 A0 | L3 L4 A0 | L1 L4 A0 | L1 A0 picked at (1.1188, 2.895) picked at (1.6528, 3.3333) bodies 6
sketch "Sketch21" plane through (0, 0, 1.15) normal (0, 0, 1) x (1, 0, 0)
  arc A0 (1.9583, 4) -> (1.0417, 4) centre (1.5, 3) ccw
  line L0 (1.9583, 4) -> (4, 4)
  line L1 (4, 4) -> (4, 3.5)
  line L2 (4, 3.5) -> (5, 3.5)
  line L3 (5, 3.5) -> (5, 5.2)
  line L4 (5, 5.2) -> (4, 5.2)
  line L5 (4, 5.2) -> (4, 4.45)
  line L6 (4, 4.45) -> (-0.3, 4.45)
  line L7 (-0.3, 4.45) -> (-0.3, 5.2)
  line L8 (-0.3, 5.2) -> (-2, 5.2)
  line L9 (-2, 5.2) -> (-2, 3.5)
  line L10 (-2, 3.5) -> (-1, 3.5)
  line L11 (-1, 3.5) -> (-1, 4)
  line L12 (-1, 4) -> (1.0417, 4)
  line L13 (-1, 4) -> (-1, 2)
  line L14 (-1, 3) -> (4, 3)
  line L15 (3.8, 3.6) -> (-0.8, 3.6)
  line L16 (-0.8, 3.6) -> (-0.8, 2.4)
  line L17 (-0.8, 2.4) -> (3.8, 2.4)
  line L18 (3.8, 2.4) -> (3.8, 3.6)
  line L19 (3.8, 3.6) -> (-0.8, 2.4) construction
  line L20 (-0.8, 3.6) -> (3.8, 2.4) construction
  point P0 (1.5, 3)
  dimension "d125" = 4.6
  dimension "d126" = 1.2
  constraint coincident L11.end L12.start
  constraint perpendicular L12 L13
  constraint midpoint L13 L14.start
  constraint perpendicular L13 L14
  constraint horizontal L15
  constraint perpendicular L15 L16
  constraint parallel L15 L17
  constraint parallel L16 L18
  constraint coincident L19 P0
  constraint coincident L20 P0
  constraint coincident P0 A0.centre
  measures "d125" distance of L16.end L17.end
  measures "d126" distance of L15.end L16.end
extrude "Extrude22" add sketch "Sketch21" against normal blind 0.4 separate body contours L14 L15 L16 L18 | L14 L16 L17 L18 makes body 7
sketch "Sketch22" plane through (0, 0, 0.75) normal (0, 0, -1) x (-1, 0, 0)
  line L0 (-3.8, 3.6) -> (-3.8, 2.4)
  line L1 (-3.8, 2.4) -> (0.8, 2.4)
  line L2 (0.8, 2.4) -> (0.8, 3.6)
  line L3 (0.8, 3.6) -> (-3.8, 3.6)
  line L4 (0.8, 2.4) -> (0.4, 2.4)
  line L5 (0.4, 2.4) -> (0.4, 3.6)
  line L6 (0.4, 3.6) -> (0.8, 3.6)
  line L7 (0.8, 3.6) -> (0.8, 2.4)
  line L8 (-3.8, 2.4) -> (-3.4, 2.4)
  line L9 (-3.4, 2.4) -> (-3.4, 3.6)
  line L10 (-3.4, 3.6) -> (-3.8, 3.6)
  line L11 (-3.8, 3.6) -> (-3.8, 2.4)
  dimension "d129" = 0.4
  dimension "d130" = 0.4
  constraint horizontal L4
  constraint vertical L5
  constraint horizontal L6
  constraint vertical L7
  constraint coincident L1.end L2.start
  constraint horizontal L8
  constraint vertical L9
  constraint horizontal L10
  constraint vertical L11
  constraint coincident L0.end L1.start
  measures "d129" distance of L1.end L4.end
  measures "d130" distance of L0.end L8.end
extrude "Extrude23" add sketch "Sketch22" along normal blind 1 contours L0 L1 L3 L8 L9 L10 L11 | L1 L2 L3 L4 L5 L6 L7 bodies 7
fillet "Fillet6" radius 0.2 2 edges at (-0.8, 3, 1.15) (3.8, 3, 1.15) on bodies 7
move_body "Move1" bodies 7 to x (0.99863, 0, 0.052336) y (0, 1, 0) z (-0.052336, 0, 0.99863) at (-0.0116, 0, -0.5084)
coil "CoilPrimitive1" add diameter 1.8 section circle size 0.2 on centre turns 8 pitch 0.35625 right hand placed x (1, 0, 0) y (0, 1, 0) z (0, 0, 1) at (1.5, 3, -2.55) separate body makes body 8
copy_body "CopyPasteBodies1" bodies 6 makes body 9
move_body "Move2" bodies 9 to x (1, 0, 0) y (0, 1, 0) z (0, 0, 1) at (0, 0, 0)
combine "Combine1" operation cut target body 8 tool bodies 9
equation "d3 = ( 19.5 / 2 ) * 1 mm"
equation "d83 = 3.8 mm - 1.1 mm"
